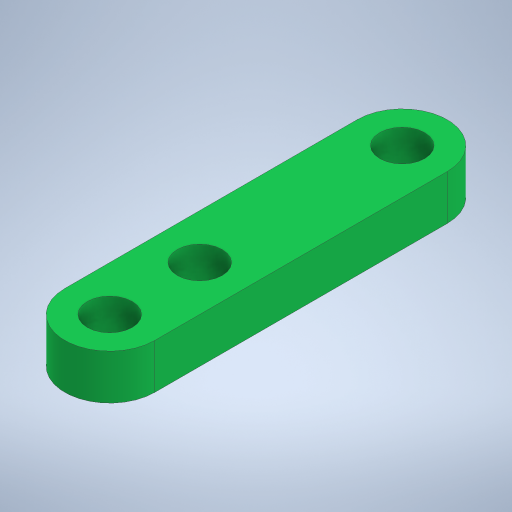
# Autodesk Inventor part: Gear to Finger Connect
Saved by Autodesk Inventor 2023.1 (Build 271208000, 208)
## iProperties
Created: 2022-11-06
Part Number: Gear to Finger Connect
Material: Generic
Document SubType Name: Modeling
Designer: shubh
Density: 1 g/cm^3
Appearance: Default
Author: shubh
Autodesk Inventor part; units mm, degrees
ref_plane "YZ Plane" through (0, 0, 0) normal (1, 0, 0) x (0, 1, 0)
ref_plane "XZ Plane" through (0, 0, 0) normal (0, 1, 0) x (-1, 0, 0)
ref_plane "XY Plane" through (0, 0, 0) normal (0, 0, 1) x (1, 0, 0)
sketch "Sketch1" plane through (0, 0, 0) normal (0, 1, 0) x (-1, 0, 0)
  circle A0 centre (0, 0) radius 3.175
  circle A1 centre (0, -12.7) radius 3.175
  line L0 (-6.35, -15.875) -> (-6.35, 0)
  line L1 (6.35, 0) -> (6.35, -15.875)
  line L2 (-6.35, 0) -> (-3.175, 0)
  line L3 (-6.35, -15.875) -> (-6.35, -41.275)
  circle A2 centre (0, -41.275) radius 3.175
  arc A3 (-6.35, -41.275) -> (6.35, -41.275) centre (0, -41.275) ccw
  line L4 (-6.35, -41.275) -> (-6.35, -15.875)
  line L5 (-6.35, -15.875) -> (0, -15.875)
  line L6 (6.35, -15.875) -> (6.35, -41.275)
  arc A4 (6.35, 0) -> (-6.35, 0) centre (0, 0) ccw
  point P0 (6.35, -7.9375)
  dimension "d0" = 6.35
  dimension "d1" = 6.35
  dimension "d14" = 6.35
  dimension "d17" = 12.7
  dimension "d18" = 6.35
  dimension "d19" = 6.35
  dimension "d20" = 12.7
  dimension "d21" = 12.7
  dimension "d22" = 12.7
  constraints: 14 end point, 4 point on circle, 3 centre point, 3 coincident, 2 parallel, 1 horizontal alignment, 1 midpoint, 1 point on line, 1 vertical alignment, 4 other
  measures "d14" diameter of A2
  measures "d17" distance from line of L0 point (6.35, -7.938)
  measures "d18" distance from line of L1 point (0, 0)
  measures "d19" distance from line of L1 point (0, -12.7)
  measures "d20" diameter of A3
  measures "d21" diameter of A4
  measures "d22" distance of point (0, 0) point (0, -12.7)
extrude "Extrusion1" add sketch "Sketch1" along normal blind 6.35
body "Solid1"
